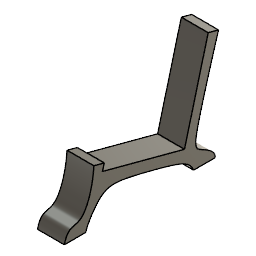
flipdot-stand (Autodesk Fusion 360 design; units mm, degrees)
Autodesk Fusion 360 part; units mm, degrees
sketch "Sketch1" plane through (0, 0, 0) normal (1, 0, 0) x (0, 1, 0)
  line L0 (-30.6201, 33.0319) -> (30.2655, 16.8473)
  line L1 (30.2655, 16.8473) -> (47.8656, 83.0578)
  line L2 (-30.6201, 33.0319) -> (-29.3356, 37.8641)
  line L3 (-29.3356, 37.8641) -> (-37.0671, 39.9192)
  line L4 (47.8656, 83.0578) -> (55.5971, 81.0026)
  spline S0 degree 5 poles (55.5971, 81.0026) (54.8835, 78.6263) (53.4911, 73.9765) (51.5067, 67.3096) (49.0703, 59.0388) (46.3801, 49.7455) (44.0559, 41.5149) (42.1124, 34.3616) (40.5672, 28.291) (39.4406, 23.291) (38.7541, 19.3234) (38.5287, 16.3145) (38.7839, 14.1424) (39.5342, 12.6279) (40.7894, 11.5126) (42.5247, 10.5195) (44.6476, 9.4254) (46.957, 8.1389) (49.1915, 6.6661) (51.0882, 5.0643) (52.4369, 3.4011) (52.9986, 2.0486) (53.1167, 1.0271) (53.0613, 0.3429) (53, 0) knots 0 0 0 0 0 0 0.05 0.1 0.15 0.2 0.25 0.3 0.35 0.4 0.45 0.5 0.55 0.6 0.65 0.7 0.75 0.8 0.85 0.9 0.95 1 1 1 1 1 1
  line L5 (53, 0) -> (37, 0)
  spline S1 degree 5 poles (-37.0671, 39.9192) (-37.1009, 39.2995) (-37.1812, 38.0602) (-37.3399, 36.2015) (-37.6286, 33.7239) (-38.1197, 30.6319) (-38.7437, 27.5562) (-39.5034, 24.5197) (-40.4009, 21.561) (-41.4372, 18.7376) (-42.6107, 16.1335) (-43.9167, 13.8508) (-45.3448, 11.982) (-46.8774, 10.5848) (-48.4878, 9.6585) (-50.1369, 9.1107) (-51.7738, 8.7503) (-53.3453, 8.3488) (-54.8032, 7.6821) (-56.1143, 6.5907) (-57.2616, 4.9898) (-58.0427, 3.2711) (-58.5513, 1.7323) (-58.8561, 0.5959) (-59, 0) knots 0 0 0 0 0 0 0.05 0.1 0.15 0.2 0.25 0.3 0.35 0.4 0.45 0.5 0.55 0.6 0.65 0.7 0.75 0.8 0.85 0.9 0.95 1 1 1 1 1 1
  line L6 (-59, 0) -> (-43, 0)
  spline S2 degree 5 poles (-43, 0) (-42.9475, 0.2542) (-42.8182, 0.7837) (-42.5518, 1.6413) (-42.0514, 2.9118) (-41.1877, 4.7037) (-40.0999, 6.6742) (-38.819, 8.7694) (-37.385, 10.9146) (-35.8352, 13.0236) (-34.1951, 15.0082) (-32.466, 16.7874) (-30.6227, 18.2939) (-28.6193, 19.4745) (-26.3935, 20.2934) (-23.8712, 20.734) (-20.9723, 20.8006) (-17.6259, 20.5137) (-13.7823, 19.9076) (-9.4274, 19.0271) (-4.5959, 17.9244) (0.6139, 16.6561) (6.0283, 15.2808) (11.4308, 13.8532) (16.589, 12.4199) (21.2864, 11.0127) (25.3459, 9.6462) (28.6713, 8.3075) (31.2494, 6.9607) (33.247, 5.5187) (34.8456, 3.9034) (35.8579, 2.4492) (36.4819, 1.262) (36.8374, 0.4278) (37, 0) knots 0 0 0 0 0 0 0.033333 0.066667 0.1 0.133333 0.166667 0.2 0.233333 0.266667 0.3 0.333333 0.366667 0.4 0.433333 0.466667 0.5 0.533333 0.566667 0.6 0.633333 0.666667 0.7 0.733333 0.766667 0.8 0.833333 0.866667 0.9 0.933333 0.966667 1 1 1 1 1 1
  line L7 (26, 10) -> (36, 4)
  point P0 (39, 14)
  point P1 (42.8399, 10.3752)
  point P2 (51, 5)
  point P3 (-41, 20)
  point P4 (-48, 10)
  point P5 (-54, 8)
  point P6 (-41, 5)
  point P7 (-35, 14)
  point P8 (-27, 20)
  point P9 (-5, 18)
  point P10 (31, 7)
  dimension "d1" = 63
  dimension "d2" = 5
  dimension "d3" = 8
  dimension "d4" = 8
  constraint perpendicular L0 L1
  constraint perpendicular L0 L2
  constraint perpendicular L2 L3
  constraint perpendicular L1 L4
  constraint horizontal L5
  constraint horizontal L6
  constraint midpoint P10 L7
  measures "d1" distance of L0.start L0.end
  measures "d2" distance of L0.start L2.end
  measures "d3" distance of L2.end L3.end
  measures "d4" distance of L1.end L4.end
extrude "Extrude1" add sketch "Sketch1" along normal blind 20
